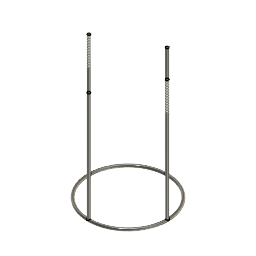
Handle_Rope_Assembly (Autodesk Fusion 360 archive; units mm, degrees)
design "Cage_ring_metal"
Autodesk Fusion 360 part; units mm, degrees
note: some values were not read from the file. Set by a fixed rule: which face or edge a step refers to.
sketch "Skizze1" plane through (0, 0, 0) normal (0, 1, 0) x (1, 0, 0)
  circle A0 centre (51.5, 0) radius 2
  dimension "d1" = 4
  dimension "d2" = 51.5
  measures "d1" diameter of A0
  measures "d2" distance of origin A0.centre
revolve "Drehen1" add sketch "Skizze1" angle 360 about axis through (0, 0, 1.75) along (0, 0, 1)
sketch "Skizze2" plane through (0, 0, 0) normal (0, 0, 1) x (1, 0, 0)
  circle A0 centre (51.5, 0) radius 2
  dimension "d4" = 4
  dimension "d5" = 51.5
  measures "d4" diameter of A0
  measures "d5" distance of origin A0.centre
extrude "Extrusion1" add sketch "Skizze2" along normal blind 160
pattern_circular "C-Anordnung1" count 4 over 360 about axis through (0, 0, 1.75) along (0, 0, 1) of "Extrusion1"
extrude "Extrusion2" cut 2 faces at (-0.65, 51.5487, 160) (0.5528, -50.3521, 160) along direction (0, 0, -1) blind 15
thread "Gewinde1" "ISO Metric profile 4.0 M4x0.7 M4x0.7 6g" major diameter 3.908 minor diameter 3.111 pitch 0.7 angle 60 resizes the face on face at (-50.9305, 1.9172, 54.6081) from (-51.5, 0, 123) to (-51.5, 0, 160) on face at (50.9304, -1.9172, 54.6081) from (51.5, 0, 123) to (51.5, 0, 160)
equation "d4 = d1"
equation "d5 = d2"
